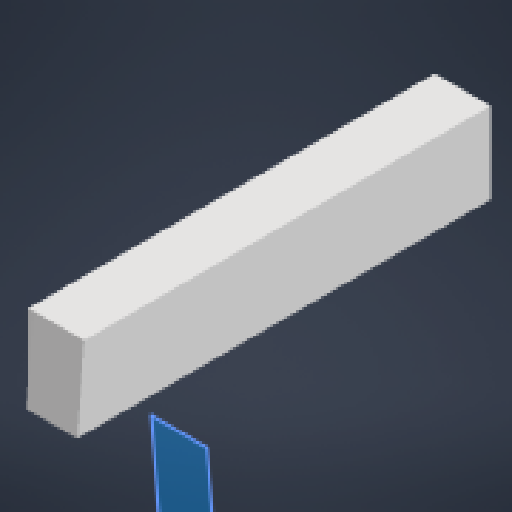
# Autodesk Inventor part: motorstand2
Saved by Autodesk Inventor 2026.2 (Build 302298000, 298)
## iProperties
Created: 2026-02-24
Part Number: motorstand2
Material: Generic
Document SubType Name: Modeling
Designer: danda
Density: 1 g/cm^3
Appearance: Default
Author: danda
Autodesk Inventor part; units mm, degrees
ref_plane "YZ Plane" through (0, 0, 0) normal (1, 0, 0) x (0, 1, 0)
ref_plane "XZ Plane" through (0, 0, 0) normal (0, 1, 0) x (-1, 0, 0)
ref_plane "XY Plane" through (0, 0, 0) normal (0, 0, 1) x (1, 0, 0)
sketch "Sketch1" plane through (0, 0, 0) normal (0, 0, 1) x (1, 0, 0)
  line L0 (22.0768, 42.8051) -> (34.0768, 42.8051)
  line L1 (34.0768, 42.8051) -> (34.0768, 20.8051)
  line L2 (34.0768, 20.8051) -> (22.0768, 20.8051)
  line L3 (22.0768, 20.8051) -> (22.0768, 42.8051)
  line L4 (39.0768, 47.8051) -> (17.0768, 47.8051)
  line L5 (17.0768, 47.8051) -> (17.0768, 15.8051)
  line L6 (17.0768, 15.8051) -> (39.0768, 15.8051)
  line L7 (39.0768, 15.8051) -> (39.0768, 47.8051)
  line L8 (34.0768, 20.8051) -> (34.0768, 15.8051)
  line L9 (22.0768, 20.8051) -> (22.0768, 15.8051)
  line L10 (22.0768, 42.8051) -> (22.0768, 47.8051)
  line L11 (34.0768, 42.8051) -> (34.0768, 47.8051)
  point P0 (0, 0)
  dimension "d4" = 12
  dimension "d5" = 22
  dimension "d6" = 5
  constraints: 24 end point, 6 point on line, 4 parallel, 4 perpendicular, 1 horizontal, 3 other
  measures "d4" distance of L1.end L2.end
  measures "d5" distance of L0.end L1.end
  measures "d6" distance between parallel lines of L0 L4
extrude "Extrusion2" add sketch "Sketch1" along normal blind 100 and the other way blind 60 contours L10 L4 L11 L0 | L3 L9 L6 L5 L4 L10 | L11 L4 L7 L6 L8 L1 | L2 L8 L6 L9
sketch "Sketch2" plane through (39.0768, 15.8051, 100) normal (1, 0, 0) x (0, 0, -1)
  line L0 (0, 0) -> (0, 32) projected
  line L1 (0, 0) -> (30.1146, 0) construction
  line L2 (0, 32) -> (-2.7996, 0)
  line L3 (0, 32) -> (32.6362, 32) construction
  line L4 (0, 0) -> (-2.7996, 0)
  point P0 (100, -15.8051)
  dimension "d16" = 95
  constraints: 8 end point, 3 horizontal
  measures "d16" angle of L2 L3
extrude "Extrusion3" add sketch "Sketch2" against normal blind 20
sketch "Sketch3" plane through (0, 0, -60) normal (0, 0, -1) x (-1, 0, 0)
  line L0 (-17.0768, 15.8051) -> (-37.0768, 15.8051)
  line L1 (-37.0768, 15.8051) -> (-37.0768, 36.9275)
  line L2 (-37.0768, 36.9275) -> (-17.0768, 36.9275)
  line L3 (-17.0768, 36.9275) -> (-17.0768, 15.8051)
  line L4 (-22.0768, 20.8051) -> (-34.0768, 20.8051)
  line L5 (-34.0768, 20.8051) -> (-34.0768, 34.8394)
  line L6 (-34.0768, 34.8394) -> (-22.0768, 34.8394)
  line L7 (-22.0768, 34.8394) -> (-22.0768, 20.8051)
  point P0 (0, 0)
  dimension "d17" = 20
  dimension "d18" = 12
  constraints: 16 end point, 4 parallel, 2 horizontal, 2 perpendicular
  measures "d17" distance of L1.end L2.end
  measures "d18" distance of L5.end L6.end
extrude "Extrusion4" add sketch "Sketch3" against normal blind 20 contours L4 L5 L6 L7
extrude "Extrusion5" cut sketch "Sketch3" against normal blind 15 contours L4 L5 L6 L7
body "Solid2"
